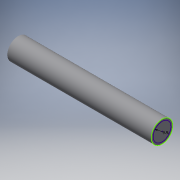
# Autodesk Inventor part: 10PI축
Saved by Autodesk Inventor 2017 (Build 210142000, 142)
## iProperties
Part Number: 10PI축
Material: 일반
Document SubType Name: Modeling
Designer: minom
Density: 1 g/cm^3
Appearance: 기본값
Author: minom
Autodesk Inventor part; units mm, degrees
ref_plane "YZ Plane" through (0, 0, 0) normal (1, 0, 0) x (0, 1, 0)
ref_plane "XZ Plane" through (0, 0, 0) normal (0, 1, 0) x (-1, 0, 0)
ref_plane "XY Plane" through (0, 0, 0) normal (0, 0, 1) x (1, 0, 0)
sketch "스케치1" plane through (0, 0, 0) normal (1, 0, 0) x (0, 1, 0)
  circle A0 centre (0, 0) radius 6
  dimension "d0" = 12
  constraints: 1 centre point, 1 coincident
  measures "d0" diameter of A0
extrude "돌출1" add sketch "스케치1" along normal blind 80
sketch "스케치2" plane through (80, 0, 0) normal (1, 0, 0) x (0, 0, -1)
  circle A0 centre (0, 0) radius 6
  circle A1 centre (0, 0) radius 4.95
  dimension "d3" = 9.9
  constraints: 2 centre point, 2 coincident
  measures "d3" diameter of A1
extrude "돌출2" cut sketch "스케치2" against normal blind 26
sketch "스케치3" plane through (80, 0, 0) normal (1, 0, 0) x (0, 0, -1)
  circle A0 centre (0, 0) radius 4.95
  circle A1 centre (0, 0) radius 4.8
  dimension "d6" = 9.9
  dimension "d7" = 9.6
  constraints: 2 centre point, 2 coincident
  measures "d6" diameter of A0
  measures "d7" diameter of A1
extrude "돌출3" cut sketch "스케치3" against normal blind 21.75
sketch "스케치4" plane through (80, 0, 0) normal (1, 0, 0) x (0, 0, -1)
  circle A0 centre (0, 0) radius 4.95
  circle A1 centre (0, 0) radius 4.8
  dimension "d10" = 9.9
  dimension "d11" = 9.6
  constraints: 2 centre point, 2 coincident
  measures "d10" diameter of A0
  measures "d11" diameter of A1
extrude "돌출4" add sketch "스케치4" against normal blind 20.65
